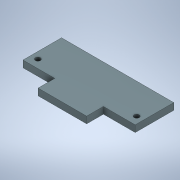
# Autodesk Inventor part: WeightFront
Saved by Autodesk Inventor 2021 (Build 250183000, 183)
## iProperties
Created: 2022-04-12
Part Number: WeightFront
Material: Lead
Document SubType Name: Modeling
Designer: ermoz
Density: 11.34 g/cm^3
Appearance: Lead
Author: ermoz
Autodesk Inventor part; units mm, degrees
ref_plane "YZ Plane" through (0, 0, 0) normal (1, 0, 0) x (0, 1, 0)
ref_plane "XZ Plane" through (0, 0, 0) normal (0, 1, 0) x (-1, 0, 0)
ref_plane "XY Plane" through (0, 0, 0) normal (0, 0, 1) x (1, 0, 0)
sketch "Sketch1" plane through (0, 0, 0) normal (0, 1, 0) x (-1, 0, 0)
  line L0 (-33.5, -11.5) -> (33.5, -11.5)
  line L1 (33.5, -11.5) -> (33.5, 11.5)
  line L2 (33.5, 11.5) -> (-33.5, 11.5)
  line L3 (-33.5, 11.5) -> (-33.5, -11.5)
  line L4 (-33.5, -11.5) -> (33.5, 11.5) construction
  line L5 (33.5, -11.5) -> (-33.5, 11.5) construction
  line L6 (-14.5, 21.5) -> (14.5, 21.5)
  line L7 (14.5, 21.5) -> (14.5, 11.5)
  line L8 (14.5, 11.5) -> (-14.5, 11.5)
  line L9 (-14.5, 11.5) -> (-14.5, 21.5)
  line L10 (-14.5, 21.5) -> (14.5, 11.5) construction
  line L11 (14.5, 21.5) -> (-14.5, 11.5) construction
  point P0 (0, 0)
  point P1 (0, 16.5)
  point P2 (0, 0)
  point P3 (0, 16.5)
  point P4 (-14.5, 11.5)
  dimension "d0" = 67
  dimension "d1" = 23
  dimension "d2" = 29
  dimension "d3" = 10
  constraints: 24 end point, 6 midpoint, 4 parallel, 2 horizontal, 2 perpendicular, 1 collinear, 1 vertical alignment
  measures "d0" distance of L0.start L0.end
  measures "d1" distance of L0.end L1.end
  measures "d2" distance of L6.start L6.end
  measures "d3" distance of L6.end L7.end
extrude "Extrusion1" add sketch "Sketch1" along normal blind 4
sketch "Sketch2" plane through (0, 4, 0) normal (0, 1, 0) x (1, 0, 0)
  circle A0 centre (-29.5, -6.625) radius 1.5
  circle A1 centre (29.5, -6.625) radius 1.5
  line L0 (33.5, -11.5) -> (33.5, 11.5) projected
  line L1 (-33.5, 11.5) -> (-33.5, -11.5) projected
  line L2 (33.5, 11.5) -> (-33.5, 11.5) projected
  point P0 (0, 0)
  dimension "d6" = 4
  dimension "d7" = 4
  dimension "d8" = 18.125
  dimension "d9" = 18.125
  dimension "d10" = 3
  constraints: 2 centre point, 1 equal radius
  measures "d6" distance from line of L0 A1.centre
  measures "d7" distance from line of L1 A0.centre
  measures "d8" distance from line of L2 A1.centre
  measures "d9" distance from line of L2 A0.centre
  measures "d10" diameter of A0
extrude "Extrusion2" cut sketch "Sketch2" against normal through all
chamfer "Chamfer1" distance 2 angle 45 2 edges at (28, 0, 6.625) (-31, 0, 6.625)
equation "\"d7\" = d6"
equation "\"d9\" = d8"
body "Solid1"
